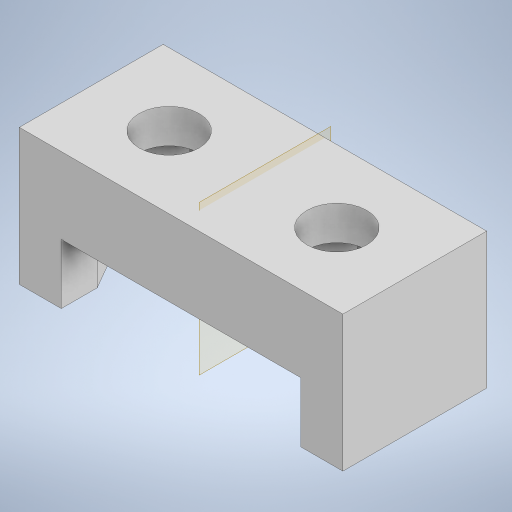
# Autodesk Inventor part: Idle Bearing mount
Saved by Autodesk Inventor 2023.1 (Build 271208000, 208)
## iProperties
Created: 2022-10-29
Part Number: Idle Bearing mount
Material: Generic
Document SubType Name: Modeling
Designer: nicol
Density: 1 g/cm^3
Appearance: Default
Author: nicol
Autodesk Inventor part; units mm, degrees
ref_plane "YZ Plane" through (0, 0, 0) normal (1, 0, 0) x (0, 1, 0)
ref_plane "XZ Plane" through (0, 0, 0) normal (0, 1, 0) x (-1, 0, 0)
ref_plane "XY Plane" through (0, 0, 0) normal (0, 0, 1) x (1, 0, 0)
sketch "Sketch1" plane through (0, 0, 0) normal (0, 0, 1) x (1, 0, 0)
  line L0 (0, 0) -> (27, 0)
  line L1 (27, 0) -> (27, 6.35)
  line L2 (27, 6.35) -> (0, 6.35)
  line L3 (0, 6.35) -> (0, 0)
  line L4 (0, 0) -> (0, -5)
  line L5 (0, -5) -> (3.5, -5)
  line L6 (3.5, -5) -> (3.5, 0)
  line L7 (27, 0) -> (27, -5)
  line L8 (27, -5) -> (23.5, -5)
  line L9 (23.5, -5) -> (23.5, 0)
  dimension "d0" = 27
  dimension "d1" = 6.35
  dimension "d14" = 20
  dimension "d15" = 5
  constraints: 20 end point, 6 perpendicular, 2 equal length, 2 parallel, 2 point on line, 1 horizontal, 1 vertical
  measures "d0" distance of L1.end L2.end
  measures "d1" distance of L0.end L1.end
  measures "d14" distance between parallel lines of L6 L9
  measures "d15" distance of L5.end L6.end
extrude "Extrusion1" add sketch "Sketch1" along normal blind 12
sketch "Sketch2" plane through (0, 6.35, 0) normal (0, 1, 0) x (1, 0, 0)
  line L0 (0, 0) -> (0, -12) projected
  line L1 (27, 0) -> (27, -12) projected
  point P0 (6.5, -6)
  point P1 (20.5, -6)
  point P2 (0, -6)
  dimension "d4" = 6.5
  dimension "d5" = 6.5
  dimension "d6" = 14
  constraints: 2 horizontal alignment, 1 midpoint
  measures "d4" distance from line of L1 point (20.5, -6)
  measures "d5" distance from line of point (6.5, -6) L0
  measures "d6" distance of point (6.5, -6) point (20.5, -6)
hole "Hole1" at (6.5, 6.35, 6) at (20.5, 6.35, 6) direction (0, -1, 0) diameter 5 end through all
sketch "Sketch3" plane through (3.5, 0, 0) normal (0, -1, 0) x (1, 0, 0)
  circle A0 centre (3, 6) radius 2.5 projected
  circle A1 centre (17, 6) radius 2.5 projected
  line L0 (0, 0) -> (20, 0) projected
  line L1 (20, 0) -> (20, 12) projected
  line L2 (0, 12) -> (20, 12) projected
  line L3 (0, 0) -> (0, 12) projected
  line L4 (7.7343, 6) -> (5.3671, 1.9)
  line L5 (5.3671, 1.9) -> (0.6329, 1.9)
  line L6 (0.6329, 1.9) -> (-1.7343, 6)
  line L7 (-1.7343, 6) -> (0.6329, 10.1)
  line L8 (0.6329, 10.1) -> (5.3671, 10.1)
  line L9 (5.3671, 10.1) -> (7.7343, 6)
  point P0 (-3.5, 0)
  point P1 (0, 9.0038)
  point P2 (0, 2.9962)
  dimension "d16" = 8.2
  constraints: 12 end point, 1 coincident, 1 horizontal, 13 other
  measures "d16" distance between parallel lines of L5 L8
extrude "Extrusion2" cut sketch "Sketch3" along normal blind 6.75 and the other way blind 3.5 contours L6 L7 L3 | L3 L7 L8 L9 L4 L5 L6
ref_plane "Work Plane1" through (13.5, -5, 0) normal (1, 0, 0) x (0, 0, -1)
mirror "Mirror1" about plane through (13.5, -5, 0) normal (1, 0, 0) of "Extrusion2"
equation "\"d5\" = d4"
body "Solid1"
